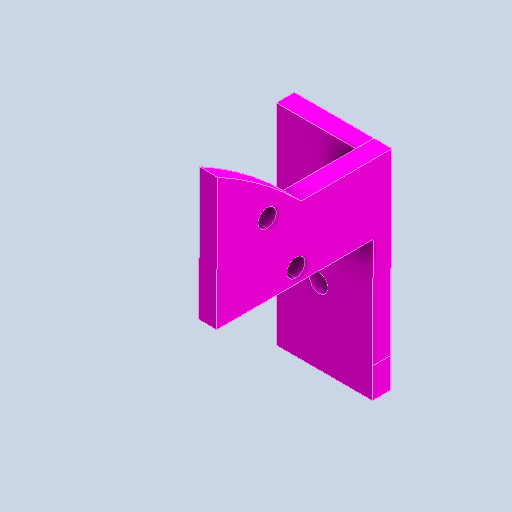
# Autodesk Inventor part: encoderholder
Saved by Autodesk Inventor 2022 (Build 260153000, 153)
## iProperties
Created: 2025-02-10
Part Number: encoderholder
Material: Типовые
Document SubType Name: Modeling
Designer: korsh624
Density: 1 g/cm^3
Appearance: Пурпурный
Author: korsh624
Autodesk Inventor part; units mm, degrees
ref_plane "YZ Plane" through (0, 0, 0) normal (1, 0, 0) x (0, 1, 0)
ref_plane "XZ Plane" through (0, 0, 0) normal (0, 1, 0) x (-1, 0, 0)
ref_plane "XY Plane" through (0, 0, 0) normal (0, 0, 1) x (1, 0, 0)
sketch "Эскиз1" plane through (0, 0, 0) normal (0, 0, 1) x (1, 0, 0)
  circle A0 centre (-3.8814, -5.2176) radius 1.5 projected
  line L0 (-10.8201, 1.8432) -> (-11.0949, -29.6556) projected
  line L1 (4.4221, -85.0622) -> (5.4693, 34.9331) projected
  line L2 (-9.8587, -12.7657) -> (-5.4656, -12.804) projected
  line L3 (-10.9475, -12.7562) -> (5.315, -12.7562)
  line L4 (5.315, -12.7562) -> (5.315, 17.2438)
  line L5 (5.315, 17.2438) -> (-10.9475, 17.2438)
  line L6 (-10.9475, 17.2438) -> (-10.9475, -12.7562)
  point P0 (0, 0)
  point P1 (5.1784, 1.5986)
  point P2 (5.0531, -12.7562)
  dimension "d0" = 30
  constraints: 8 end point, 2 parallel, 2 point on line, 1 horizontal, 1 perpendicular, 1 other
  measures "d0" distance of L4.end L3.end
extrude "Выдавливание1" add sketch "Эскиз1" along normal blind 3 contours L3 L6 L5 L1
sketch "Эскиз2" plane through (5.315, 17.2438, 3) normal (0.9999619, -0.0087265, 0) x (0, 0, -1)
  spline S0 degree 3 poles (-15.9024, -10.7583) (-16.7308, -10.7583) (-17.4024, -10.0867) (-17.4024, -9.2583) (-17.4024, -8.4299) (-16.7308, -7.7583) (-15.9024, -7.7583) (-15.074, -7.7583) (-14.4024, -8.4299) (-14.4024, -9.2583) (-14.4024, -10.0867) (-15.074, -10.7583) (-15.9024, -10.7583) knots 0 0 0 0 0.25 0.25 0.25 0.5 0.5 0.5 0.75 0.75 0.75 1 1 1 1 projected
  spline S1 degree 3 poles (-20.7708, -1.1274) (-21.5992, -1.1274) (-22.2708, -0.4558) (-22.2708, 0.3726) (-22.2708, 1.201) (-21.5992, 1.8726) (-20.7708, 1.8726) (-19.9424, 1.8726) (-19.2708, 1.201) (-19.2708, 0.3726) (-19.2708, -0.4558) (-19.9424, -1.1274) (-20.7708, -1.1274) knots 0 0 0 0 0.25 0.25 0.25 0.5 0.5 0.5 0.75 0.75 0.75 1 1 1 1 projected
  line L0 (0, -30.0011) -> (0, 0) projected
  line L1 (0, -11.6364) -> (-29.1176, -11.6364)
  spline S2 degree 3 poles (-117.3896, -48.1529) (-114.4523, -78.5481) (-88.8364, -102.3099) (-57.6706, -102.3099) (-24.5335, -102.3099) (2.3293, -75.4471) (2.3293, -42.31) (2.3293, -9.1729) (-24.5335, 17.69) (-57.6706, 17.69) (-89.3782, 17.69) (-115.3412, -6.9053) (-117.5222, -38.0583) knots 0 0 0 0 0.2 0.2 0.2 0.4 0.4 0.4 0.6 0.6 0.6 0.8 0.8 0.8 0.8 projected
  line L2 (-29.1176, -11.6364) -> (-29.1176, 10.4736)
  line L3 (-15.1281, 0) -> (0, 0)
  point P0 (3, -17.2895)
  point P1 (-15.9024, -10.7583)
  point P2 (-20.7708, -1.1274)
  constraints: 6 end point, 1 horizontal, 1 perpendicular, 1 point on line, 1 vertical, 2 other
extrude "Выдавливание2" add sketch "Эскиз2" against normal blind 3 contours L1 S2 L3 L0 | L1 L2 S2
sketch "Эскиз3" plane through (0, 0, 0) normal (0, 0, -1) x (-1, 0, 0)
  line L0 (-5.315, 17.2438) -> (10.9475, 17.2438) projected
  line L1 (10.9475, -12.7562) -> (-5.0531, -12.7562) projected
  line L2 (10.9475, 17.2438) -> (10.9475, -12.7562) projected
  line L3 (-5.315, 17.2438) -> (10.9475, 17.2438) projected
  line L4 (-5.0531, -12.7562) -> (-5.315, 17.2438) projected
  circle A0 centre (3.8814, -5.2176) radius 1.5 projected
  point P0 (0, 0)
extrude "Выдавливание3" add sketch "Эскиз3" against normal blind 6
sketch "Эскиз4" plane through (0, 0, 0) normal (0, 0, -1) x (-1, 0, 0)
  line L0 (10.9475, -12.7562) -> (-5.0531, -12.7562) projected
  line L1 (10.9475, 17.2438) -> (10.9475, -12.7562) projected
  line L2 (-5.315, 17.2438) -> (10.9475, 17.2438) projected
  line L3 (-5.0531, -12.7562) -> (-5.315, 17.2438) projected
  circle A0 centre (3.8814, -5.2176) radius 1.5 projected
  point P0 (0, 0)
extrude "Выдавливание4" cut sketch "Эскиз4" against normal blind 3
sketch "Эскиз5" plane through (-10.9475, -12.7562, 3) normal (0, -1, 0) x (1, 0, 0)
  line L0 (0, 0) -> (16.0006, 0) projected
  line L1 (16.0006, 0) -> (16.0006, 3) projected
  line L2 (0, 3) -> (16.0006, 3) projected
  line L3 (0, 0) -> (0, 3) projected
  point P0 (10.9475, -3)
extrude "Выдавливание5" add sketch "Эскиз5" along normal blind 5
